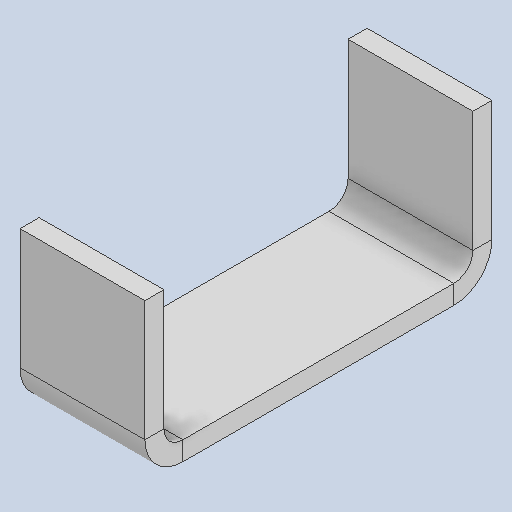
# Autodesk Inventor part: bracket1-01
Saved by Autodesk Inventor 2022 (Build 260153000, 153)
## iProperties
Created: 2022-04-22
Part Number: bracket1-01
Material: Generic
Document SubType Name: Sheet Metal
Designer: HP
Density: 1 g/cm^3
Sheet Metal Rule: Default
Appearance: Default
Author: HP
Autodesk Inventor part; units mm, degrees
ref_plane "YZ Plane" through (0, 0, 0) normal (1, 0, 0) x (0, 1, 0)
ref_plane "XZ Plane" through (0, 0, 0) normal (0, 1, 0) x (-1, 0, 0)
ref_plane "XY Plane" through (0, 0, 0) normal (0, 0, 1) x (1, 0, 0)
sketch "Sketch1" plane through (0, 0, 0) normal (0, 1, 0) x (-1, 0, 0)
  line L0 (10, 27.8) -> (-10, 27.8)
  line L1 (-10, 27.8) -> (-10, -27.8)
  line L2 (-10, -27.8) -> (10, -27.8)
  line L3 (10, -27.8) -> (10, 27.8)
  line L4 (10, 27.8) -> (-10, -27.8) construction
  line L5 (-10, 27.8) -> (10, -27.8) construction
  point P0 (0, 0)
  dimension "d0" = 55.6
  dimension "d1" = 20
  measures "d0" distance of L2.end L0.start
  measures "d1" distance of L1.end L2.end
extrude "Plate1" add sketch "Sketch1" along normal blind 3.048
sketch "Sketch2" plane through (10, 0, 27.8) normal (0, 0, -1) x (-1, 0, 0)
  line L0 (20, 3.048) -> (0, 3.048)
  line L1 (0, 3.048) -> (0, 25.4)
  line L2 (0, 25.4) -> (20, 25.4)
  line L3 (20, 25.4) -> (20, 3.048)
  constraints: 8 end point
edge flange "Flange1" height 25.4 angle 90 thickness 3.048 bend radius 3.048 thickness toward (0, 0, -1) relief tear relief width 3.048 relief depth 1.524 edges at (0, 3.048, 27.8) wall of the first edge with corners at (-10, 3.048, 27.8) (10, 3.048, 27.8) (10, 25.4, 27.8) (-10, 25.4, 27.8)
bend "Bend1"
corner "Corner1"
sketch "Sketch3" plane through (-10, 0, -27.8) normal (0, 0, 1) x (1, 0, 0)
  line L0 (20, 3.048) -> (0, 3.048)
  line L1 (0, 3.048) -> (0, 25.4)
  line L2 (0, 25.4) -> (20, 25.4)
  line L3 (20, 25.4) -> (20, 3.048)
  constraints: 8 end point
edge flange "Flange2" height 25.4 angle 90 thickness 3.048 bend radius 3.048 thickness toward (0, 0, 1) relief tear relief width 3.048 relief depth 1.524 edges at (0, 3.048, -27.8) wall of the first edge with corners at (10, 3.048, -27.8) (-10, 3.048, -27.8) (-10, 25.4, -27.8) (10, 25.4, -27.8)
bend "Bend2"
corner "Corner2"
equation "\"d2\" = Thickness"
equation "\"d3\" = BendReliefWidth"
equation "\"d4\" = BendReliefDepth"
equation "\"d5\" = MinimumRemnant"
equation "\"d6\" = TransitionRadius"
equation "\"d9\" = BendRadius"
equation "\"d10\" = CornerReliefSize"
equation "\"d11\" = GapSize"
equation "\"d12\" = JacobiRadiusSize"
equation "\"d13\" = BendReliefWidth"
equation "\"d14\" = BendReliefDepth"
equation "\"d15\" = MinimumRemnant"
equation "\"d16\" = TransitionRadius"
equation "\"d19\" = BendRadius"
equation "\"d20\" = CornerReliefSize"
equation "\"d21\" = GapSize"
equation "\"d22\" = JacobiRadiusSize"
equation "\"BendRadius\" = Thickness"
equation "\"BendReliefWidth\" = Thickness"
equation "\"BendReliefDepth\" = 0.5 * Thickness"
equation "\"CornerReliefSize\" = 4 * Thickness"
equation "\"MinimumRemnant\" = 2 * Thickness"
equation "\"TransitionRadius\" = BendRadius"
equation "\"JacobiRadiusSize\" = BendRadius"
equation "\"GapSize\" = Thickness"
equation "\"Thickness\" = 3.048"
body "Solid1"
